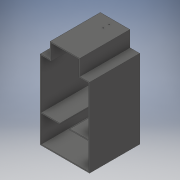
# Autodesk Inventor part: Space
Saved by Autodesk Inventor 2019 (Build 230136000, 136)
## iProperties
Created: 2019-03-04
Part Number: Space
Material: 일반
Document SubType Name: Modeling
Designer: Jeong Ji Hoon
Density: 1 g/cm^3
Appearance: 기본값
Author: Jeong Ji Hoon
Autodesk Inventor part; units mm, degrees
ref_plane "YZ Plane" through (0, 0, 0) normal (1, 0, 0) x (0, 1, 0)
ref_plane "XZ Plane" through (0, 0, 0) normal (0, 1, 0) x (-1, 0, 0)
ref_plane "XY Plane" through (0, 0, 0) normal (0, 0, 1) x (1, 0, 0)
sketch "스케치1" plane through (0, 0, 0) normal (0, 0, 1) x (1, 0, 0)
  line L0 (0, 0) -> (0, 800)
  line L1 (0, 800) -> (100, 800)
  line L2 (100, 800) -> (100, 960)
  line L3 (100, 960) -> (400, 960)
  line L4 (400, 960) -> (400, 800)
  line L5 (400, 800) -> (500, 800)
  line L6 (500, 800) -> (500, 0)
  line L7 (500, 0) -> (0, 0)
  line L8 (390, 950) -> (110, 950)
  line L9 (110, 950) -> (110, 790)
  line L10 (110, 790) -> (10, 790)
  line L11 (10, 790) -> (10, 10)
  line L12 (10, 10) -> (490, 10)
  line L13 (490, 10) -> (490, 790)
  line L14 (490, 790) -> (390, 790)
  line L15 (390, 790) -> (390, 950)
  line L16 (10, 280) -> (200, 280)
  line L17 (200, 280) -> (200, 290)
  line L18 (200, 290) -> (10, 290)
  line L19 (10, 290) -> (10, 280)
  line L20 (490, 280) -> (300, 280)
  line L21 (300, 280) -> (300, 290)
  line L22 (300, 290) -> (490, 290)
  line L23 (490, 290) -> (490, 280)
  dimension "d0" = 800
  dimension "d1" = 100
  dimension "d2" = 160
  dimension "d3" = 300
  dimension "d4" = 160
  dimension "d5" = 100
  dimension "d6" = 800
  dimension "d7" = 10
  dimension "d8" = 190
  dimension "d9" = 10
  dimension "d10" = 190
  dimension "d11" = 10
  dimension "d12" = 500
  constraints: 48 end point, 10 perpendicular, 5 point on line, 4 parallel, 2 horizontal, 1 vertical, 7 other
  measures "d0" distance of L0.start L0.end
  measures "d1" distance of L0.end L1.end
  measures "d2" distance of L1.end L2.end
  measures "d3" distance of L2.end L3.end
  measures "d4" distance of L3.end L4.end
  measures "d5" distance of L4.end L5.end
  measures "d6" distance of L5.end L6.end
  measures "d7" distance between parallel lines of L3 L8
  measures "d8" distance of L18.end L17.end
  measures "d9" distance of L17.end L16.end
  measures "d10" distance of L21.end L22.end
  measures "d11" distance of L20.end L21.end
  measures "d12" distance between parallel lines of L18 L10
extrude "돌출1" add sketch "스케치1" along normal blind 500 contours L0 L1 L2 L3 L4 L5 L6 L7 | L13 L20 L21 L22 | L18 L17 L16 L11
sketch "스케치2" plane through (0, 0, 0) normal (0, 0, -1) x (-1, 0, 0)
  line L0 (-390, 790) -> (-390, 950) projected
  line L1 (-390, 950) -> (-110, 950) projected
  line L2 (-110, 950) -> (-110, 790) projected
  line L3 (-110, 790) -> (-10, 790) projected
  line L4 (-10, 790) -> (-10, 290) projected
  line L5 (-200, 290) -> (-10, 290) projected
  line L6 (-200, 280) -> (-200, 290) projected
  line L7 (-10, 280) -> (-200, 280) projected
  line L8 (-10, 280) -> (-10, 10) projected
  line L9 (-10, 10) -> (-490, 10) projected
  line L10 (-490, 10) -> (-490, 280) projected
  line L11 (-300, 280) -> (-490, 280) projected
  line L12 (-300, 290) -> (-300, 280) projected
  line L13 (-490, 290) -> (-300, 290) projected
  line L14 (-490, 290) -> (-490, 790) projected
  line L15 (-490, 790) -> (-390, 790) projected
  line L16 (0, 0) -> (0, 800) projected
  line L17 (0, 800) -> (-100, 800) projected
  line L18 (-100, 800) -> (-100, 960) projected
  line L19 (-100, 960) -> (-400, 960) projected
  line L20 (-400, 960) -> (-400, 800) projected
  line L21 (-400, 800) -> (-500, 800) projected
  line L22 (-500, 800) -> (-500, 0) projected
  line L23 (-500, 0) -> (0, 0) projected
extrude "돌출2" add sketch "스케치2" along normal blind 10 contours L0 L1 L2 L3 L4 L5 L6 L7 L8 L9 L10 L11 L12 L13 L14 L15 | L23 L22 L21 L20 L19 L18 L17 L16
sketch "스케치4" plane through (110, 950, 500) normal (0, -1, 0) x (1, 0, 0)
  line L0 (-10, 0) -> (-10, -510) projected
  line L1 (290, 0) -> (290, -510) projected
  line L2 (-10, -510) -> (290, -510) projected
  point P0 (-110, -500)
  point P1 (140, -390)
  point P2 (140, -450)
  dimension "d18" = 150
  dimension "d28" = 60
  dimension "d29" = 120
  measures "d18" distance from line of L0 point (140, -390)
  measures "d28" distance from line of L2 point (140, -450)
  measures "d29" distance from line of L2 point (140, -390)
hole "구멍1" at (250, 950, 110) at (250, 950, 50) direction (0, 1, 0) diameter 10 end through all
